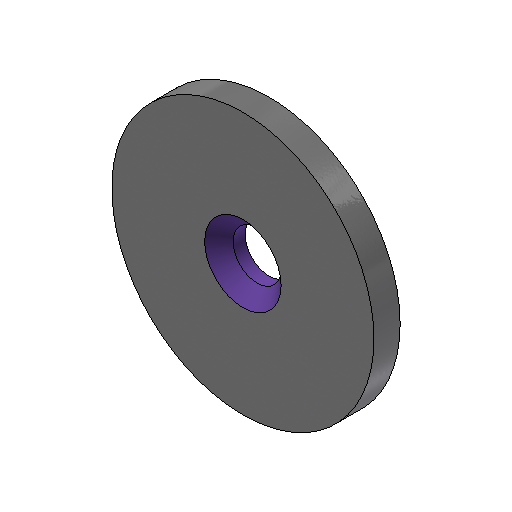
# Autodesk Inventor part: TL20240701-10110CV-019
Saved by Autodesk Inventor 2022.5 (Build 265521000, 521)
## iProperties
Category: DRIVE UNIT ASSY
Company: 현대 트랜시스(대유)
Created: 2023-04-10
Part Number: TL20240701-10110CV-019
Checked By: 김형민
Engr Approved By: 김시현
User Status: 1 x18
Material: SS400
Description: 0
Document SubType Name: Modeling
Mfg Approved By: 호상태
Designer: 박성규
Stock Number: 019
Density: 7.85 g/cm^3
Appearance: Plating Zinc White
Project: SW PJT
DETAIL: Coveryor Assembly
M/C TITLE: CJ 제일제당 협동로봇 포장시스탬 PILOT 장비
PARTS NAME: Bracket
SPECIFICATION: TA20221101-CV200000-015
DocNumber: 221118_Standard_v1
Folder: .\
VDS_Category: 엔지니어링
Detail Description: Processed products
Title: END CAP
Subject: SW차종 시트조립라인
Author: 박성규
Revision Number: A
Autodesk Inventor part; units mm, degrees
ref_plane "YZ Plane" through (0, 0, 0) normal (1, 0, 0) x (0, 1, 0)
ref_plane "XZ Plane" through (0, 0, 0) normal (0, 1, 0) x (-1, 0, 0)
ref_plane "XY Plane" through (0, 0, 0) normal (0, 0, 1) x (1, 0, 0)
sketch "스케치9" plane through (0, 0, 0) normal (0, 0, 1) x (1, 0, 0)
  circle A0 centre (0, 0) radius 30
  dimension "d40" = 60
  constraints: 1 centre point, 1 coincident
  measures "d40" diameter of A0
extrude "돌출4" add sketch "스케치9" along normal blind 6
sketch "스케치10" plane through (0, 0, 6) normal (0, 0, 1) x (1, 0, 0)
  circle A0 centre (0, 0) radius 30 construction
  constraints: 1 coincident
hole "구멍3" at (0, 0, 6) direction (0, 0, -1) diameter 11 end through all countersink diameter 17.5 countersink angle 90 clearance for "Countersunk Flat Head Screw ISO 2009/7046" size "M10" standard "ISO"
